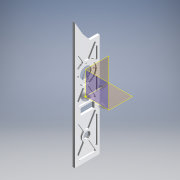
# Autodesk Inventor part: 옆판_오른쪽
Saved by Autodesk Inventor 2017 (Build 210142000, 142)
## iProperties
Part Number: 옆판_오른쪽
Material: 알루미늄 6061
Document SubType Name: Modeling
Designer: minom
Density: 2.7 g/cm^3
Appearance: 알루미늄 - 평지
Mass: 116.482 g
Surface Area: 317.94 cm^2
Volume: 43.1416 cm^3
Author: minom
Autodesk Inventor part; units mm, degrees
ref_plane "YZ Plane" through (0, 0, 0) normal (1, 0, 0) x (0, 1, 0)
ref_plane "XZ Plane" through (0, 0, 0) normal (0, 1, 0) x (-1, 0, 0)
ref_plane "XY Plane" through (0, 0, 0) normal (0, 0, 1) x (1, 0, 0)
sketch "스케치1" plane through (0, 0, 0) normal (1, 0, 0) x (0, 1, 0)
  line L0 (0, 0) -> (0, 280)
  line L1 (0, 280) -> (55, 280)
  line L2 (55, 280) -> (55, 0)
  line L3 (55, 0) -> (0, 0)
  line L4 (0, 280) -> (0, 250)
  line L5 (0, 250) -> (0, 230)
  line L6 (0, 230) -> (0, 220)
  line L7 (0, 230) -> (55, 230)
  line L8 (0, 250) -> (55, 250)
  line L9 (0, 280) -> (17.3205, 250)
  line L10 (0, 280) -> (34.641, 280) construction
  line L11 (17.3205, 250) -> (34.1025, 230)
  line L12 (17.3205, 250) -> (43.4287, 250) construction
  line L13 (34.1025, 230) -> (47.1107, 230) construction
  point P0 (55, 220)
  dimension "d0" = 280
  dimension "d1" = 55
  dimension "d2" = 30
  dimension "d3" = 20
  dimension "d5" = 60
  dimension "d6" = 50
  constraints: 28 end point, 8 point on line, 5 perpendicular, 3 horizontal, 2 equal length, 1 vertical
  measures "d0" distance of L0.start L0.end
  measures "d1" distance of L0.end L1.end
  measures "d2" distance of L0.end L4.end
  measures "d3" distance of L4.end L5.end
  measures "d5" angle of L9 L10
  measures "d6" angle of L11 L12
extrude "돌출1" add sketch "스케치1" along normal blind 5 contours L0 L7 L2 L3 | L0 L8 L11 L7 | L0 L9 L8
sketch "스케치4" plane through (5, 0, 0) normal (1, 0, 0) x (0, 0, -1)
  line L0 (-250, 17.3205) -> (-280, 0) projected
  line L1 (-280, 0) -> (-170, 0)
  line L2 (-280, 0) -> (0, 0) projected
  circle A0 centre (-169.35, 27) radius 21.25
  line L3 (0, 0) -> (0, 55) projected
  line L4 (0, 0) -> (-169.35, 0)
  line L5 (-169.35, 0) -> (-169.35, 27)
  line L6 (-169.35, 27) -> (-169.35, 0)
  dimension "d14" = 110
  dimension "d16" = 42.5
  dimension "d43" = 169.35
  dimension "d44" = 0
  constraints: 8 end point, 2 perpendicular, 2 point on line, 1 centre point
  measures "d14" distance of L0.end L1.end
  measures "d16" diameter of A0
  measures "d43" distance of L2.end L4.end
  measures "d44" distance from line of A0.centre L5
extrude "돌출2" cut sketch "스케치4" against normal blind 3
sketch "스케치5" plane through (2, 27, 169.35) normal (1, 0, 0) x (0, 0, -1)
  circle A0 centre (0, 0) radius 12.6
  point P0 (169.35, -27)
  dimension "d19" = 25.2
  constraints: 1 centre point
  measures "d19" diameter of A0
extrude "돌출3" cut sketch "스케치5" against normal blind 3
sketch "스케치6" plane through (2, 27, 169.35) normal (1, 0, 0) x (0, 0, -1)
  circle A0 centre (0, 0) radius 21.25 projected
  circle A1 centre (0, 17.6) radius 2.1
  circle A2 centre (17.6, 0) radius 2.1
  circle A3 centre (0, -17.6) radius 2.1
  circle A4 centre (-17.6, 0) radius 2.1
  point P0 (169.35, -27)
  dimension "d31" = 4.2
  dimension "d32" = 4.2
  dimension "d33" = 4.2
  dimension "d34" = 4.2
  constraints: 4 centre point
  measures "d31" diameter of A1
  measures "d32" diameter of A2
  measures "d33" diameter of A3
  measures "d34" diameter of A4
extrude "돌출4" cut sketch "스케치6" against normal blind 3 contours A1 | A2 | A3 | A4
sketch "스케치7" plane through (0, 0, 0) normal (-1, 0, 0) x (0, 0, 1)
  line L0 (280, 0) -> (0, 0) projected
  line L1 (0, 0) -> (50, 0)
  line L2 (50, 0) -> (50, 27)
  line L3 (50, 27) -> (169.35, 27)
  circle A0 centre (50, 27) radius 7.55
  dimension "d37" = 50
  dimension "d38" = 27
  dimension "d39" = 119.35
  dimension "d40" = 15.1
  constraints: 6 end point, 2 perpendicular, 1 centre point, 1 coincident, 1 point on line
  measures "d37" distance of L0.end L1.end
  measures "d38" distance of L1.end L2.end
  measures "d39" distance of L2.end L3.end
  measures "d40" diameter of A0
extrude "돌출5" cut sketch "스케치7" against normal blind 5
sketch "스케치8" plane through (5, 0, 0) normal (1, 0, 0) x (0, 0, -1)
  circle A0 centre (-50, 27) radius 7.55 projected
  circle A1 centre (-169.35, 27) radius 21.25 projected
  line L0 (-230, 34.1025) -> (-250, 17.3205) projected
  line L1 (-250, 17.3205) -> (-280, 0) projected
  line L2 (-280, 0) -> (0, 0) projected
  line L3 (0, 0) -> (0, 55) projected
  line L4 (0, 55) -> (-230, 55) projected
  line L5 (-230, 55) -> (-230, 34.1025) projected
  line L6 (0, 55) -> (-230, 55) projected
  line L7 (0, 0) -> (0, 55) projected
  line L8 (-280, 0) -> (0, 0) projected
  line L9 (-250, 17.3205) -> (-280, 0) projected
  line L10 (-169.35, 27) -> (-109.35, 27)
  line L11 (-109.35, 27) -> (-109.35, 42)
  line L12 (-109.35, 27) -> (-109.35, 14)
  line L13 (-94.35, 27) -> (-50, 27)
  line L14 (-94.35, 14) -> (-94.35, 42)
  line L15 (-108.35, 43) -> (-95.35, 43)
  line L16 (-108.35, 13) -> (-95.35, 13)
  arc A2 (-108.35, 43) -> (-109.35, 42) centre (-108.35, 42) ccw
  arc A3 (-94.35, 42) -> (-95.35, 43) centre (-95.35, 42) ccw
  arc A4 (-95.35, 13) -> (-94.35, 14) centre (-95.35, 14) ccw
  arc A5 (-109.35, 14) -> (-108.35, 13) centre (-108.35, 14) ccw
  point P0 (-109.35, 43)
  point P1 (-109.35, 13)
  point P2 (-94.35, 13)
  point P3 (-94.35, 43)
  dimension "d118" = 60
  dimension "d119" = 15
  dimension "d120" = 30
  dimension "d121" = 12
  dimension "d124" = 1
  constraints: 14 end point, 9 point on line, 8 point on circle, 8 tangent, 4 centre point, 3 equal radius, 2 perpendicular, 1 horizontal
  measures "d118" distance of L10.start L10.end
  measures "d119" distance of L10.end L13.start
  measures "d120" distance of point (-109.35, 43) point (-109.35, 13)
  measures "d121" distance between parallel lines of L15 L4
  measures "d124" radius of A2
sketch "스케치9" plane through (5, 0, 0) normal (1, 0, 0) x (0, 0, -1)
  circle A0 centre (-50, 27) radius 7.55 projected
  circle A1 centre (-169.35, 27) radius 21.25 projected
  line L0 (-230, 34.1025) -> (-250, 17.3205) projected
  line L1 (-250, 17.3205) -> (-280, 0) projected
  line L2 (-280, 0) -> (0, 0) projected
  line L3 (0, 0) -> (0, 55) projected
  line L4 (0, 55) -> (-230, 55) projected
  line L5 (-230, 55) -> (-230, 34.1025) projected
  line L6 (0, 55) -> (-230, 55) projected
  line L7 (-280, 0) -> (0, 0) projected
  line L8 (-250, 17.3205) -> (-280, 0) projected
  line L9 (-94.35, 12.641) -> (-94.35, 42.641) projected
  line L10 (0, 0) -> (0, 55) projected
  line L11 (-280, 0) -> (0, 0) projected
  line L12 (-113.35, 27.5224) -> (-113.4532, 44.2388)
  line L13 (-113.35, 27.5224) -> (-113.35, 10.7735)
  line L14 (-129.5762, 38.3819) -> (-116.4531, 45.9585)
  line L15 (-129.5762, 38.3819) -> (-143.16, 30.5393)
  line L16 (-131.5762, 13.154) -> (-142.6869, 19.5687)
  line L17 (-131.5762, 13.154) -> (-123.9172, 8.7321)
  line L18 (-129.4731, 16.6181) -> (-143.1111, 24.492)
  line L19 (-129.4731, 16.6181) -> (-116.35, 9.0415)
  line L20 (-131.5762, 41.846) -> (-142.9954, 35.2532)
  line L21 (-131.5762, 41.846) -> (-123.9172, 46.2679)
  line L22 (-90.35, 27.5224) -> (-90.35, 44.1669)
  line L23 (-90.35, 27.5224) -> (-90.35, 10.8331)
  line L24 (-78.989, 50) -> (-55.4656, 50) construction
  line L25 (-78.989, 5) -> (-55.9099, 5) construction
  line L26 (-10, 5) -> (24.1299, 5) construction
  line L27 (-10, 50) -> (24.5913, 50) construction
  line L28 (-230, 36) -> (-222, 36)
  line L29 (-222, 36) -> (-222, 10.7735)
  line L30 (-222, 36) -> (-222, 44.2265)
  line L31 (-222, 50) -> (-189.3275, 50) construction
  line L32 (-222, 5) -> (-187.8584, 5) construction
  line L33 (-204.7919, 42.3743) -> (-195.0602, 36.7557)
  line L34 (-204.7919, 42.3743) -> (-211.5359, 46.2679)
  line L35 (-206.7919, 38.9102) -> (-195.3638, 32.3122)
  line L36 (-206.7919, 38.9102) -> (-219, 45.9585)
  line L37 (-208.9634, 14.8361) -> (-219, 9.0415)
  line L38 (-208.9634, 14.8361) -> (-195.4716, 22.6256)
  line L39 (-206.9634, 11.372) -> (-195.4146, 18.0397)
  line L40 (-206.9634, 11.372) -> (-211.5359, 8.7321)
  arc A2 (-219, 45.9585) -> (-222, 44.2265) centre (-220, 44.2265) ccw
  arc A3 (-222, 10.7735) -> (-219, 9.0415) centre (-220, 10.7735) ccw
  arc A4 (-211.5359, 8.7321) -> (-210.5359, 5) centre (-210.5359, 7) ccw
  arc A5 (-210.5359, 50) -> (-211.5359, 46.2679) centre (-210.5359, 48) ccw
  arc A6 (-123.9172, 46.2679) -> (-124.9172, 50) centre (-124.9172, 48) ccw
  arc A7 (-113.4532, 44.2388) -> (-116.4531, 45.9585) centre (-115.4531, 44.2265) ccw
  arc A8 (-116.35, 9.0415) -> (-113.35, 10.7735) centre (-115.35, 10.7735) ccw
  arc A9 (-124.9172, 5) -> (-123.9172, 8.7321) centre (-124.9172, 7) ccw
  arc A10 (-192.575, 17.0924) -> (-186.5, 8.4679) centre (-169.35, 27) ccw
  arc A11 (-194.3811, 30.3174) -> (-194.481, 24.5516) centre (-169.35, 27) ccw
  arc A12 (-185.441, 46.4587) -> (-192.2466, 37.6446) centre (-169.35, 27) ccw
  arc A13 (-145.8563, 36.2524) -> (-153.259, 46.4587) centre (-169.35, 27) ccw
  arc A14 (-144.1102, 26.281) -> (-144.1556, 28.6746) centre (-169.35, 27) ccw
  line L41 (-124.9172, 50) -> (-151.9844, 50)
  line L42 (-186.7156, 50) -> (-210.5359, 50)
  arc A15 (-152.2, 8.4679) -> (-145.5704, 18.5092) centre (-169.35, 27) ccw
  line L43 (-124.9172, 5) -> (-150.8416, 5)
  arc A16 (-194.3811, 30.3174) -> (-195.3638, 32.3122) centre (-196.3638, 30.5801) ccw
  arc A17 (-195.4716, 22.6256) -> (-194.481, 24.5516) centre (-196.4716, 24.3576) ccw
  arc A18 (-192.575, 17.0924) -> (-195.4146, 18.0397) centre (-194.4146, 16.3076) ccw
  arc A19 (-187.8584, 5) -> (-186.5, 8.4679) centre (-187.8584, 7) ccw
  arc A20 (-195.0602, 36.7557) -> (-192.2466, 37.6446) centre (-194.0602, 38.4878) ccw
  arc A21 (-185.441, 46.4587) -> (-186.7156, 50) centre (-186.7156, 48) ccw
  arc A22 (-151.9844, 50) -> (-153.259, 46.4587) centre (-151.9844, 48) ccw
  arc A23 (-145.8563, 36.2524) -> (-142.9954, 35.2532) centre (-143.9954, 36.9852) ccw
  arc A24 (-143.16, 30.5393) -> (-144.1556, 28.6746) centre (-142.16, 28.8073) ccw
  arc A25 (-144.1102, 26.281) -> (-143.1111, 24.492) centre (-142.1111, 26.224) ccw
  arc A26 (-142.6869, 19.5687) -> (-145.5704, 18.5092) centre (-143.6869, 17.8367) ccw
  arc A27 (-152.2, 8.4679) -> (-150.8416, 5) centre (-150.8416, 7) ccw
  line L44 (-210.5359, 5) -> (-187.8584, 5)
  line L45 (-73.9594, 38.1679) -> (-62.2798, 31.4247)
  line L46 (-73.9594, 38.1679) -> (-87.35, 45.899)
  line L47 (-71.9594, 41.632) -> (-60.4446, 34.984)
  line L48 (-71.9594, 41.632) -> (-79.989, 46.2679)
  line L49 (-71.9594, 13.368) -> (-61.0636, 19.6587)
  line L50 (-71.9594, 13.368) -> (-79.989, 8.7321)
  line L51 (-73.9594, 16.8321) -> (-62.4325, 23.4871)
  line L52 (-73.9594, 16.8321) -> (-87.35, 9.101)
  line L53 (-28.4938, 13.368) -> (-39.0933, 19.4876)
  line L54 (-28.4938, 13.368) -> (-20.4641, 8.7321)
  line L55 (-26.4938, 16.8321) -> (-37.6018, 23.2453)
  line L56 (-26.4938, 16.8321) -> (-13, 9.0415)
  line L57 (-28.4938, 41.632) -> (-39.7261, 35.147)
  line L58 (-28.4938, 41.632) -> (-20.4641, 46.2679)
  line L59 (-26.4938, 38.1679) -> (-37.7696, 31.6578)
  line L60 (-26.4938, 38.1679) -> (-13, 45.9585)
  line L61 (-78.989, 5) -> (-21.4641, 5)
  line L62 (-10, 27.5) -> (-10, 10.7735)
  line L63 (-10, 27.5) -> (-10, 44.2265)
  line L64 (-78.989, 50) -> (-21.4641, 50)
  arc A28 (-61.3197, 29.2952) -> (-61.4498, 25.482) centre (-50, 27) ccw
  arc A29 (-58.5782, 19.2659) -> (-41.5555, 19.1201) centre (-50, 27) ccw
  arc A30 (-38.5794, 25.2759) -> (-38.7225, 29.4939) centre (-50, 27) ccw
  arc A31 (-42.0949, 35.4209) -> (-58.0506, 35.2819) centre (-50, 27) ccw
  arc A32 (-87.35, 45.899) -> (-90.35, 44.1669) centre (-88.35, 44.1669) ccw
  arc A33 (-61.3197, 29.2952) -> (-62.2798, 31.4247) centre (-63.2798, 29.6926) ccw
  arc A34 (-62.4325, 23.4871) -> (-61.4498, 25.482) centre (-63.4325, 25.2192) ccw
  arc A35 (-90.35, 10.8331) -> (-87.35, 9.101) centre (-88.35, 10.8331) ccw
  arc A36 (-58.5782, 19.2659) -> (-61.0636, 19.6587) centre (-60.0636, 17.9266) ccw
  arc A37 (-39.0933, 19.4876) -> (-41.5555, 19.1201) centre (-40.0933, 17.7556) ccw
  arc A38 (-21.4641, 5) -> (-20.4641, 8.7321) centre (-21.4641, 7) ccw
  arc A39 (-79.989, 8.7321) -> (-78.989, 5) centre (-78.989, 7) ccw
  arc A40 (-78.989, 50) -> (-79.989, 46.2679) centre (-78.989, 48) ccw
  arc A41 (-60.4446, 34.984) -> (-58.0506, 35.2819) centre (-59.4446, 36.716) ccw
  arc A42 (-42.0949, 35.4209) -> (-39.7261, 35.147) centre (-40.7261, 36.8791) ccw
  arc A43 (-20.4641, 46.2679) -> (-21.4641, 50) centre (-21.4641, 48) ccw
  arc A44 (-10, 44.2265) -> (-13, 45.9585) centre (-12, 44.2265) ccw
  arc A45 (-13, 9.0415) -> (-10, 10.7735) centre (-12, 10.7735) ccw
  arc A46 (-38.5794, 25.2759) -> (-37.6018, 23.2453) centre (-36.6018, 24.9774) ccw
  arc A47 (-37.7696, 31.6578) -> (-38.7225, 29.4939) centre (-36.7696, 29.9257) ccw
  point P0 (-230, 50)
  point P1 (-268.4206, 6.6853)
  point P2 (-144.2671, 29.9002)
  point P3 (-144.8662, 20.8269)
  point P4 (-117.4531, 5)
  point P5 (-144.1713, 25.1041)
  point P6 (-113.35, 7.3094)
  point P7 (-145.1006, 34.0377)
  point P8 (-90.35, 5)
  point P9 (-193.0848, 35.6152)
  point P10 (-218, 50)
  point P11 (-194.1729, 31.6246)
  point P12 (-222, 47.6906)
  point P13 (-194.3255, 23.2873)
  point P14 (-193.3713, 19.2194)
  point P15 (-218, 5)
  point P16 (-179.7693, 50)
  point P17 (-158.9307, 50)
  point P18 (-156.958, 5)
  point P19 (-60.9549, 30.6597)
  point P20 (-59.0487, 34.178)
  point P21 (-59.564, 20.5245)
  point P22 (-61.2045, 24.1961)
  point P23 (-40.5653, 20.3375)
  point P24 (-14, 5)
  point P25 (-38.8549, 23.9688)
  point P26 (-10, 7.3094)
  point P27 (-41.0957, 34.3563)
  point P28 (-14, 50)
  point P29 (-39.1205, 30.8779)
  point P30 (-10, 47.6906)
  point P31 (-90.35, 47.631)
  point P32 (-90.35, 7.369)
  dimension "d83" = 4
  dimension "d91" = 8
  dimension "d95" = 4
  dimension "d97" = 4
  dimension "d98" = 2
  dimension "d99" = 2
  dimension "d101" = 4
  dimension "d107" = 2
  dimension "d117" = 4
  constraints: 111 point on circle, 106 end point, 75 tangent, 60 point on line, 46 centre point, 33 equal radius, 9 horizontal, 9 parallel, 6 coincident, 2 perpendicular, 1 collinear
  measures "d83" distance of L20.start L14.start
  measures "d91" distance of L28.start L28.end
  measures "d95" distance of L39.start L37.start
  measures "d97" distance of L35.start L33.start
  measures "d98" radius of A2
  measures "d99" radius of A16
  measures "d101" distance of L47.start L45.start
  measures "d107" radius of A32
  measures "d117" radial gap between concentric circles of A1 A14
extrude "돌출7" cut sketch "스케치9" against normal blind 3 contours L13 A8 L19 L18 A25 A14 A24 L15 L14 A7 L12 | L17 A9 L43 A27 A15 A26 L16 | L20 A23 A13 A22 L41 A6 L21 | L22 A32 L46 L45 A33 A28 A34 L51 L52 A35 L23 | L30 A2 L36 L35 A16 A11 A17 L38 L37 A3 L29 | L34 A5 L42 A21 A12 A20 L33 | L39 A18 A10 A19 L44 A4 L40 | L48 A40 L64 A43 L58 L57 A42 A31 A41 L47 | L49 A36 A29 A37 L53 L54 A38 L61 A39 L50 | L55 A46 A30 A47 L59 L60 A44 L63 L62 A45 L56
extrude "돌출8" cut sketch "스케치8" against normal blind 5 contours L11 A2 L15 A3 L14 A4 L16 A5 L12
